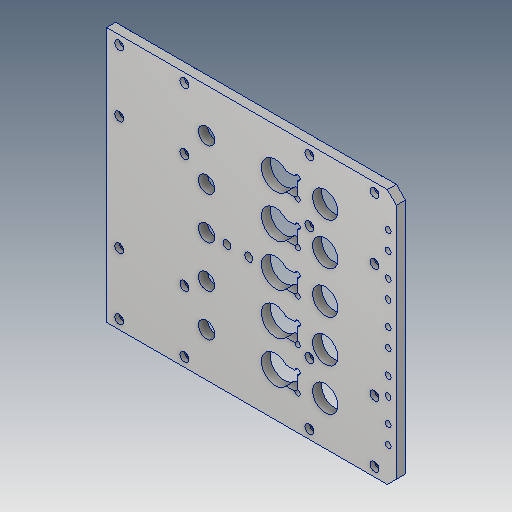
# Autodesk Inventor part: bottom-plate
Saved by Autodesk Inventor 2017 (Build 210142000, 142)
## iProperties
Created: 2018-06-17
Part Number: bottom-plate
Material: Aluminum 6061
Document SubType Name: Sheet Metal
Designer: Luiz Gustavo
Density: 2.7 g/cm^3
Sheet Metal Rule: Default_mm
Appearance: Aluminum - Flat
Author: Luiz Gustavo
Autodesk Inventor part; units mm, degrees
ref_plane "YZ Plane" through (0, 0, 0) normal (1, 0, 0) x (0, 1, 0)
ref_plane "XZ Plane" through (0, 0, 0) normal (0, 1, 0) x (-1, 0, 0)
ref_plane "XY Plane" through (0, 0, 0) normal (0, 0, 1) x (1, 0, 0)
sketch "Sketch1" plane through (0, 0, 0) normal (0, 0, 1) x (1, 0, 0)
  line L0 (-37.3, 70.5) -> (-32.3, 70.5) construction
  line L1 (-37.3, 52.15) -> (-37.3, 70.5) construction
  arc A0 (-37.3, 40.65) -> (-37.3, 52.15) centre (-37.3, 46.4) ccw construction
  line L2 (-37.3, 28.95) -> (-37.3, 40.65) construction
  arc A1 (-37.3, 17.45) -> (-37.3, 28.95) centre (-37.3, 23.2) ccw construction
  line L3 (-37.3, 5.75) -> (-37.3, 17.45) construction
  arc A2 (-37.3, -5.75) -> (-37.3, 5.75) centre (-37.3, 0) ccw construction
  line L4 (-37.3, -17.45) -> (-37.3, -5.75) construction
  arc A3 (-37.3, -28.95) -> (-37.3, -17.45) centre (-37.3, -23.2) ccw construction
  line L5 (-37.3, -40.65) -> (-37.3, -28.95) construction
  arc A4 (-37.3, -52.15) -> (-37.3, -40.65) centre (-37.3, -46.4) ccw construction
  line L6 (-37.3, -52.15) -> (-37.3, -70.5) construction
  line L7 (-37.3, -70.5) -> (-32.3, -70.5) construction
  circle A5 centre (24.95, -51.4) radius 2.05 construction
  circle A6 centre (24.95, -28.2) radius 2.05 construction
  circle A7 centre (24.95, -5) radius 2.05 construction
  circle A8 centre (24.95, 18.2) radius 2.05 construction
  circle A9 centre (24.95, 41.4) radius 2.05 construction
  line L8 (-23.6527, -42.9) -> (-20.4, -42.9) construction
  line L9 (-20.4, -42.9) -> (-20.4, -36.3) construction
  line L10 (-20.4, -36.3) -> (20.4, -36.3) construction
  line L11 (20.4, -36.3) -> (20.4, -56.5) construction
  line L12 (20.4, -56.5) -> (-20.4, -56.5) construction
  line L13 (-20.4, -56.5) -> (-20.4, -49.9) construction
  line L14 (-20.4, -49.9) -> (-23.6527, -49.9) construction
  arc A10 (-26.4473, -49.9) -> (-23.6527, -49.9) centre (-25.05, -51.4) ccw construction
  line L15 (-28.4, -49.9) -> (-28.4, -42.9) construction
  arc A11 (-23.6527, -42.9) -> (-26.4473, -42.9) centre (-25.05, -41.4) ccw construction
  line L16 (-23.6527, -19.7) -> (-20.4, -19.7) construction
  line L17 (-20.4, -19.7) -> (-20.4, -13.1) construction
  line L18 (-20.4, -13.1) -> (20.4, -13.1) construction
  line L19 (20.4, -13.1) -> (20.4, -33.3) construction
  line L20 (20.4, -33.3) -> (-20.4, -33.3) construction
  line L21 (-20.4, -33.3) -> (-20.4, -26.7) construction
  line L22 (-20.4, -26.7) -> (-23.6527, -26.7) construction
  arc A12 (-26.4473, -26.7) -> (-23.6527, -26.7) centre (-25.05, -28.2) ccw construction
  line L23 (-28.4, -26.7) -> (-28.4, -19.7) construction
  arc A13 (-23.6527, -19.7) -> (-26.4473, -19.7) centre (-25.05, -18.2) ccw construction
  line L24 (-23.6527, 3.5) -> (-20.4, 3.5) construction
  line L25 (-20.4, 3.5) -> (-20.4, 10.1) construction
  line L26 (-20.4, 10.1) -> (20.4, 10.1) construction
  line L27 (20.4, 10.1) -> (20.4, -10.1) construction
  line L28 (20.4, -10.1) -> (-20.4, -10.1) construction
  line L29 (-20.4, -10.1) -> (-20.4, -3.5) construction
  line L30 (-20.4, -3.5) -> (-23.6527, -3.5) construction
  arc A14 (-26.4473, -3.5) -> (-23.6527, -3.5) centre (-25.05, -5) ccw construction
  line L31 (-28.4, -3.5) -> (-28.4, 3.5) construction
  arc A15 (-23.6527, 3.5) -> (-26.4473, 3.5) centre (-25.05, 5) ccw construction
  line L32 (-23.6527, 26.7) -> (-20.4, 26.7) construction
  line L33 (-20.4, 26.7) -> (-20.4, 33.3) construction
  line L34 (-20.4, 33.3) -> (20.4, 33.3) construction
  line L35 (20.4, 33.3) -> (20.4, 13.1) construction
  line L36 (20.4, 13.1) -> (-20.4, 13.1) construction
  line L37 (-20.4, 13.1) -> (-20.4, 19.7) construction
  line L38 (-20.4, 19.7) -> (-23.6527, 19.7) construction
  arc A16 (-26.4473, 19.7) -> (-23.6527, 19.7) centre (-25.05, 18.2) ccw construction
  line L39 (-28.4, 19.7) -> (-28.4, 26.7) construction
  arc A17 (-23.6527, 26.7) -> (-26.4473, 26.7) centre (-25.05, 28.2) ccw construction
  line L40 (-23.6527, 49.9) -> (-20.4, 49.9) construction
  line L41 (-20.4, 49.9) -> (-20.4, 56.5) construction
  line L42 (-20.4, 56.5) -> (20.4, 56.5) construction
  line L43 (20.4, 56.5) -> (20.4, 36.3) construction
  line L44 (20.4, 36.3) -> (-20.4, 36.3) construction
  line L45 (-20.4, 36.3) -> (-20.4, 42.9) construction
  line L46 (-20.4, 42.9) -> (-23.6527, 42.9) construction
  arc A18 (-26.4473, 42.9) -> (-23.6527, 42.9) centre (-25.05, 41.4) ccw construction
  line L47 (-28.4, 42.9) -> (-28.4, 49.9) construction
  arc A19 (-23.6527, 49.9) -> (-26.4473, 49.9) centre (-25.05, 51.4) ccw construction
  circle A20 centre (24.95, 51.4) radius 2.05 construction
  circle A21 centre (24.95, 28.2) radius 2.05 construction
  circle A22 centre (24.95, 5) radius 2.05 construction
  circle A23 centre (24.95, -18.2) radius 2.05 construction
  circle A24 centre (24.95, -41.4) radius 2.05 construction
  line L48 (29.5, -70.5) -> (-130.5, -70.5)
  line L49 (-130.5, -70.5) -> (-130.5, 70.5)
  line L50 (-130.5, 70.5) -> (29.5, 70.5)
  line L51 (29.5, 70.5) -> (29.5, -70.5)
  circle A25 centre (24.95, -51.4) radius 1.65
  circle A26 centre (24.95, -41.4) radius 1.65
  circle A27 centre (24.95, -28.2) radius 1.65
  circle A28 centre (24.95, -18.2) radius 1.65
  circle A29 centre (24.95, -5) radius 1.65
  circle A30 centre (24.95, 5) radius 1.65
  circle A31 centre (24.95, 18.2) radius 1.65
  circle A32 centre (24.95, 28.2) radius 1.65
  circle A33 centre (24.95, 41.4) radius 1.65
  circle A34 centre (24.95, 51.4) radius 1.65
  circle A35 centre (-25.05, 51.4) radius 1.5
  circle A36 centre (-25.05, 41.4) radius 1.5
  circle A37 centre (-25.05, 28.2) radius 1.5
  circle A38 centre (-25.05, 18.2) radius 1.5
  circle A39 centre (-25.05, 5) radius 1.5
  circle A40 centre (-25.05, -5) radius 1.5
  circle A41 centre (-25.05, -18.2) radius 1.5
  circle A42 centre (-25.05, -28.2) radius 1.5
  circle A43 centre (-25.05, -51.4) radius 1.5
  circle A44 centre (-25.05, -41.4) radius 1.5
  circle A45 centre (-37.3, -46.4) radius 7.75
  circle A46 centre (-37.3, -23.2) radius 7.75
  circle A47 centre (-37.3, 0) radius 7.75
  circle A48 centre (-37.3, 23.2) radius 7.75
  circle A49 centre (-37.3, 46.4) radius 7.75
  line L52 (-37.3, -46.4) -> (-9.8, -46.4) construction
  circle A50 centre (-9.8, -46.4) radius 7
  line L53 (-37.3, 46.4) -> (-9.8, 46.4) construction
  line L54 (-9.8, 46.4) -> (-9.8, -46.4) construction
  line L55 (-37.3, 23.2) -> (-9.8, 23.2) construction
  line L56 (-37.3, -23.2) -> (-9.8, -23.2) construction
  line L57 (-37.3, 0) -> (-9.8, 0) construction
  circle A51 centre (-9.8, -23.2) radius 7
  circle A52 centre (-9.8, 0) radius 7
  circle A53 centre (-9.8, 23.2) radius 7
  circle A54 centre (-9.8, 46.4) radius 7
  circle A55 centre (-75.3, -46.4) radius 4.5
  line L58 (-37.3, -46.4) -> (-45.05, -46.4) construction
  line L59 (-37.3, 46.4) -> (-75.3, 46.4) construction
  line L60 (-75.3, 46.4) -> (-75.3, -46.4) construction
  line L61 (-37.3, -23.2) -> (-75.3, -23.2) construction
  line L62 (-37.3, 0) -> (-75.3, 0) construction
  line L63 (-37.3, 23.2) -> (-75.3, 23.2) construction
  circle A56 centre (-75.3, -23.2) radius 4.5
  circle A57 centre (-75.3, 0) radius 4.5
  circle A58 centre (-75.3, 23.2) radius 4.5
  circle A59 centre (-75.3, 46.4) radius 4.5
  line L64 (-45.05, -46.4) -> (-70.8, -46.4) construction
  line L65 (-70.8, -46.4) -> (-75.3, -46.4) construction
  circle A60 centre (-87.5161, -31.5337) radius 2.5 projected
  circle A61 centre (-87.5838, 31.2662) radius 2.5 projected
  circle A62 centre (-123.5838, 31.2274) radius 2.5 projected
  circle A63 centre (-123.5161, -31.5725) radius 2.5 projected
  arc A64 (-206.8064, -40.6623) -> (-200.7999, -46.6558) centre (-200.8064, -40.6558) ccw projected
  line L66 (-206.8064, -40.6623) -> (-206.8934, 40.1377) projected
  arc A65 (-200.8999, 46.1441) -> (-206.8934, 40.1377) centre (-200.8934, 40.1441) ccw projected
  line L67 (-40.4, 46.3171) -> (-200.8999, 46.1441) projected
  arc A66 (-40.4, 46.3171) -> (-34.4, 46.3235) centre (-37.4, 46.3203) ccw projected
  line L68 (-19.9, 46.3392) -> (-34.4, 46.3235) projected
  arc A67 (0.1, 46.3607) -> (-19.9, 46.3392) centre (-9.9, 46.3499) ccw projected
  line L69 (0.2, -46.4392) -> (0.1, 46.3607) projected
  arc A68 (-19.8, -46.4608) -> (0.2, -46.4392) centre (-9.8, -46.45) ccw projected
  line L70 (-19.8, -46.4608) -> (-34.3, -46.4764) projected
  arc A69 (-34.3, -46.4764) -> (-40.3, -46.4829) centre (-37.3, -46.4796) ccw projected
  line L71 (-40.3, -46.4829) -> (-200.7999, -46.6558) projected
  arc A70 (-190.8268, -21.6451) -> (-195.8268, -21.6504) centre (-193.3268, -21.6478) ccw projected
  line L72 (-195.8268, -21.6504) -> (-195.8161, -31.6504) projected
  arc A71 (-195.8161, -31.6504) -> (-190.8161, -31.6451) centre (-193.3161, -31.6477) ccw projected
  line L73 (-190.8161, -31.6451) -> (-190.8268, -21.6451) projected
  arc A72 (-190.8837, 31.1549) -> (-195.8837, 31.1495) centre (-193.3837, 31.1522) ccw projected
  line L74 (-195.8837, 31.1495) -> (-195.873, 21.1495) projected
  arc A73 (-195.873, 21.1495) -> (-190.873, 21.1549) centre (-193.373, 21.1522) ccw projected
  line L75 (-190.873, 21.1549) -> (-190.8837, 31.1549) projected
  arc A74 (-165.8837, 31.1819) -> (-170.8837, 31.1765) centre (-168.3837, 31.1792) ccw projected
  line L76 (-170.8837, 31.1765) -> (-170.873, 21.1765) projected
  arc A75 (-170.873, 21.1765) -> (-165.873, 21.1819) centre (-168.373, 21.1792) ccw projected
  line L77 (-165.873, 21.1819) -> (-165.8837, 31.1819) projected
  circle A76 centre (-37.375, 23.1203) radius 3 projected
  circle A77 centre (-37.325, -23.2796) radius 3 projected
  circle A78 centre (-37.35, -0.0797) radius 3 projected
  arc A79 (-178.373, 21.1684) -> (-183.373, 21.163) centre (-180.873, 21.1657) ccw projected
  line L78 (-183.373, 21.163) -> (-183.3622, 11.163) projected
  arc A80 (-183.3622, 11.163) -> (-178.3622, 11.1684) centre (-180.8622, 11.1657) ccw projected
  line L79 (-178.3622, 11.1684) -> (-178.373, 21.1684) projected
  arc A81 (-178.3376, -11.6316) -> (-183.3376, -11.637) centre (-180.8376, -11.6343) ccw projected
  line L80 (-183.3376, -11.637) -> (-183.3268, -21.637) projected
  arc A82 (-183.3268, -21.637) -> (-178.3268, -21.6316) centre (-180.8268, -21.6343) ccw projected
  line L81 (-178.3268, -21.6316) -> (-178.3376, -11.6316) projected
  arc A83 (-165.8268, -21.6181) -> (-170.8268, -21.6235) centre (-168.3268, -21.6208) ccw projected
  line L82 (-170.8268, -21.6235) -> (-170.8161, -31.6235) projected
  arc A84 (-170.8161, -31.6235) -> (-165.8161, -31.6181) centre (-168.3161, -31.6208) ccw projected
  line L83 (-165.8161, -31.6181) -> (-165.8268, -21.6181) projected
  circle A85 centre (-9.9, 46.3499) radius 1.1 projected
  circle A86 centre (-9.875, 23.15) radius 1.1 projected
  circle A87 centre (-9.8, -46.45) radius 1.1 projected
  circle A88 centre (-9.825, -23.25) radius 1.1 projected
  circle A89 centre (-9.85, -0.05) radius 1.1 projected
  line L84 (-26.4473, 42.9) -> (-28.4, 42.9) projected
  line L85 (-28.4, 49.9) -> (-26.4473, 49.9) projected
  line L86 (-26.4473, -3.5) -> (-28.4, -3.5) projected
  line L87 (-28.4, 3.5) -> (-26.4473, 3.5) projected
  line L88 (-26.4473, -49.9) -> (-28.4, -49.9) projected
  line L89 (-28.4, -42.9) -> (-26.4473, -42.9) projected
  line L90 (-26.4473, -26.7) -> (-28.4, -26.7) projected
  line L91 (-28.4, -19.7) -> (-26.4473, -19.7) projected
  line L92 (-26.4473, 19.7) -> (-28.4, 19.7) projected
  line L93 (-28.4, 26.7) -> (-26.4473, 26.7) projected
  line L94 (29, 61.5) -> (-23.3, 61.5) projected
  arc A90 (-32.3, 70.5) -> (-23.3, 61.5) centre (-23.3, 70.5) ccw projected
  arc A91 (-23.3, -61.5) -> (-32.3, -70.5) centre (-23.3, -70.5) ccw projected
  line L95 (-23.3, -61.5) -> (29, -61.5) projected
  line L96 (29, -61.5) -> (29, 61.5) projected
  point P0 (0, 0)
  dimension "d2" = 15.5
  dimension "d5" = 9
  dimension "d0" = 160
  dimension "d3" = 27.5
  dimension "d4" = 14
  dimension "d6" = 38
  dimension "d28" = 25.75
  dimension "d78" = 3
  dimension "d79" = 3.3
  constraints: 36 end point, 33 centre point, 28 equal radius, 24 coincident, 9 horizontal, 4 perpendicular, 4 point on line, 2 collinear, 2 horizontal alignment, 2 midpoint, 2 parallel, 1 vertical, 6 other
  measures "d0" distance between parallel lines of L49 L51
  measures "d3" distance of L52.start L52.end
  measures "d4" diameter of A50
  measures "d6" distance of L52.start L60.end
  measures "d28" distance of L58.end L64.end
  measures "d78" diameter of A35
  measures "d79" diameter of A34
extrude "Plate1" add sketch "Sketch1" along normal blind 5 contours L48 A91 L95 L96 L94 A90 L50 L51 | L48 L49 L71 A55 A45 L70 A68 L69 A67 L68 A49 L67 A59 L50 A90 L94 L96 L95 A91 | L49 L67 A59 A49 L68 A67 L69 A68 L70 A45 L71 A55 | A60 | A61 | A62 | A63
sketch "Sketch2" plane through (0, 0, 0) normal (0, 0, 1) x (1, 0, 0)
  line L0 (24.5, -70.5) -> (-25.5, -70.5) construction
  line L1 (-25.5, -70.5) -> (-25.5, -26.5) construction
  line L2 (-25.5, -26.5) -> (24.5, -26.5) construction
  line L3 (24.5, -26.5) -> (24.5, -70.5) construction
  circle A0 centre (-18.5, -65.5) radius 2.5
  circle A1 centre (17.5, -65.5) radius 2.5
  circle A2 centre (17.5, -31.5) radius 2.5
  circle A3 centre (-18.5, -31.5) radius 2.5
  line L4 (-18.5, -65.5) -> (17.5, -65.5) construction
  line L5 (17.5, -65.5) -> (17.5, -31.5) construction
  line L6 (17.5, -31.5) -> (-18.5, -31.5) construction
  line L7 (-18.5, -31.5) -> (-18.5, -65.5) construction
  line L8 (-12.7, -31.5) -> (-12.7, -65.5) construction
  line L9 (11.7, -31.5) -> (11.7, -65.5) construction
  line L10 (29.5, -70.5) -> (-130.5, -70.5) construction
  line L11 (-130.5, -70.5) -> (-130.5, 70.5) construction
  line L12 (29.5, 70.5) -> (29.5, -70.5) construction
  line L13 (-130.5, 70.5) -> (29.5, 70.5) construction
  line L14 (-80.5, -70.5) -> (-130.5, -70.5) construction
  line L15 (-130.5, -70.5) -> (-130.5, -26.5) construction
  line L16 (-130.5, -26.5) -> (-80.5, -26.5) construction
  line L17 (-80.5, -26.5) -> (-80.5, -70.5) construction
  circle A4 centre (-123.5, -65.5) radius 2.5
  circle A5 centre (-87.5, -65.5) radius 2.5
  circle A6 centre (-87.5, -31.5) radius 2.5
  circle A7 centre (-123.5, -31.5) radius 2.5
  line L18 (-123.5, -65.5) -> (-87.5, -65.5) construction
  line L19 (-87.5, -65.5) -> (-87.5, -31.5) construction
  line L20 (-87.5, -31.5) -> (-123.5, -31.5) construction
  line L21 (-123.5, -31.5) -> (-123.5, -65.5) construction
  line L22 (-117.7, -31.5) -> (-117.7, -65.5) construction
  line L23 (-93.3, -31.5) -> (-93.3, -65.5) construction
  line L24 (-123.5, 31.5) -> (-87.5, 31.5) construction
  line L25 (-87.5, 65.5) -> (-123.5, 65.5) construction
  line L26 (-130.5, 70.5) -> (-80.5, 70.5) construction
  line L27 (-117.7, 65.5) -> (-117.7, 31.5) construction
  line L28 (-123.5, 65.5) -> (-123.5, 31.5) construction
  circle A8 centre (-123.5, 65.5) radius 2.5
  line L29 (-130.5, 26.5) -> (-130.5, 70.5) construction
  circle A9 centre (-123.5, 31.5) radius 2.5
  line L30 (-93.3, 65.5) -> (-93.3, 31.5) construction
  circle A10 centre (-87.5, 31.5) radius 2.5
  line L31 (-87.5, 31.5) -> (-87.5, 65.5) construction
  circle A11 centre (-87.5, 65.5) radius 2.5
  line L32 (-80.5, 70.5) -> (-80.5, 26.5) construction
  line L33 (-80.5, 26.5) -> (-130.5, 26.5) construction
  line L34 (-18.5, 31.5) -> (17.5, 31.5) construction
  line L35 (17.5, 65.5) -> (-18.5, 65.5) construction
  line L36 (-25.5, 70.5) -> (24.5, 70.5) construction
  line L37 (-12.7, 65.5) -> (-12.7, 31.5) construction
  line L38 (-18.5, 65.5) -> (-18.5, 31.5) construction
  circle A12 centre (-18.5, 65.5) radius 2.5
  line L39 (-25.5, 26.5) -> (-25.5, 70.5) construction
  circle A13 centre (-18.5, 31.5) radius 2.5
  line L40 (11.7, 65.5) -> (11.7, 31.5) construction
  circle A14 centre (17.5, 31.5) radius 2.5
  line L41 (17.5, 31.5) -> (17.5, 65.5) construction
  circle A15 centre (17.5, 65.5) radius 2.5
  line L42 (24.5, 70.5) -> (24.5, 26.5) construction
  line L43 (24.5, 26.5) -> (-25.5, 26.5) construction
  point P0 (0, 0)
  dimension "d8" = 44
  dimension "d9" = 50
  dimension "d10" = 5
  dimension "d11" = 5
  dimension "d12" = 7
  dimension "d13" = 5
  dimension "d14" = 7
  dimension "d15" = 24.4
  dimension "d16" = 12.8
  dimension "d17" = 0
  dimension "d18" = 5
  dimension "d19" = 44
  dimension "d20" = 50
  dimension "d21" = 5
  dimension "d22" = 5
  dimension "d23" = 7
  dimension "d24" = 5
  dimension "d25" = 7
  dimension "d26" = 24.4
  dimension "d27" = 12.8
  dimension "d30" = 0
  dimension "d31" = 0
  dimension "d32" = 44
  dimension "d33" = 50
  dimension "d34" = 5
  dimension "d35" = 5
  dimension "d36" = 7
  dimension "d37" = 5
  dimension "d38" = 7
  dimension "d39" = 24.4
  dimension "d40" = 12.8
  dimension "d41" = 44
  dimension "d42" = 50
  dimension "d43" = 5
  dimension "d44" = 5
  dimension "d45" = 7
  dimension "d46" = 5
  dimension "d47" = 7
  dimension "d48" = 24.4
  dimension "d49" = 12.8
  dimension "d50" = 0
  dimension "d51" = 0
  dimension "d52" = 5
  dimension "d53" = 0
  constraints: 80 end point, 20 parallel, 16 centre point, 16 point on line, 12 coincident, 12 equal radius, 12 perpendicular, 8 horizontal
  measures "d8" distance of L2.end L0.start
  measures "d9" distance between parallel lines of L1 L3
  measures "d10" diameter of A0
  measures "d11" distance between parallel lines of L4 L0
  measures "d12" distance between parallel lines of L1 L7
  measures "d13" distance between parallel lines of L2 L6
  measures "d14" distance between parallel lines of L3 L5
  measures "d15" distance between parallel lines of L9 L8
  measures "d16" distance between parallel lines of L1 L8
  measures "d17" distance between parallel lines of L10 L0
  measures "d18" distance between parallel lines of L12 L3
  measures "d19" distance of L16.end L17.end
  measures "d20" distance between parallel lines of L15 L17
  measures "d21" diameter of A4
  measures "d22" distance between parallel lines of L18 L14
  measures "d23" distance between parallel lines of L15 L21
  measures "d24" distance between parallel lines of L16 L20
  measures "d25" distance between parallel lines of L17 L19
  measures "d26" distance between parallel lines of L23 L22
  measures "d27" distance between parallel lines of L15 L22
  measures "d30" distance between parallel lines of L10 L14
  measures "d31" distance between parallel lines of L11 L15
  measures "d32" distance of L26.end L33.start
  measures "d33" distance between parallel lines of L29 L32
  measures "d34" diameter of A9
  measures "d35" distance between parallel lines of L24 L33
  measures "d36" distance between parallel lines of L29 L28
  measures "d37" distance between parallel lines of L26 L25
  measures "d38" distance between parallel lines of L32 L31
  measures "d39" distance between parallel lines of L30 L27
  measures "d40" distance between parallel lines of L29 L27
  measures "d41" distance of L36.end L43.start
  measures "d42" distance between parallel lines of L39 L42
  measures "d43" diameter of A13
  measures "d44" distance between parallel lines of L34 L43
  measures "d45" distance between parallel lines of L39 L38
  measures "d46" distance between parallel lines of L36 L35
  measures "d47" distance between parallel lines of L42 L41
  measures "d48" distance between parallel lines of L40 L37
  measures "d49" distance between parallel lines of L39 L37
  measures "d50" distance between parallel lines of L26 L13
  measures "d51" distance between parallel lines of L11 L29
  measures "d52" distance between parallel lines of L12 L42
  measures "d53" distance between parallel lines of L13 L36
hole "Hole1" at (-123.5, 65.5, 0) at (-123.5, 31.5, 0) at (-87.5, 65.5, 0) at (-87.5, 31.5, 0) at (-123.5, -31.5, 0) at (-123.5, -65.5, 0) at (-87.5, -65.5, 0) at (-87.5, -31.5, 0) at (-18.5, -65.5, 0) at (17.5, -65.5, 0) at (17.5, -31.5, 0) at (-18.5, -31.5, 0) at (-18.5, 31.5, 0) at (-18.5, 65.5, 0) at (17.5, 65.5, 0) at (17.5, 31.5, 0) direction (0, 0, 1) diameter 5 end through all countersink diameter 10 countersink angle 90
sketch "Sketch3" plane through (0, 0, 0) normal (0, 0, 1) x (1, 0, 0)
  line L0 (-47.5, -20) -> (-56.5, -20)
  line L1 (-56.5, -20) -> (-56.5, 20)
  line L2 (-56.5, 20) -> (-47.5, 20)
  line L3 (-47.5, 20) -> (-47.5, -20)
  line L4 (-59.5, 20) -> (-68.5, 20)
  line L5 (-68.5, 20) -> (-68.5, -20)
  line L6 (-68.5, -20) -> (-59.5, -20)
  line L7 (-59.5, -20) -> (-59.5, 20)
  line L8 (-47.5, 0) -> (-68.5, 0) construction
  line L9 (-64, 20) -> (-64, -20) construction
  line L10 (-52, 20) -> (-52, -20) construction
  circle A0 centre (-64, 0) radius 2
  circle A1 centre (-52, 0) radius 2
  line L11 (-130.5, 70.5) -> (29.5, 70.5) projected
  line L12 (-130.5, -70.5) -> (-130.5, 70.5) projected
  line L13 (29.5, -70.5) -> (-130.5, -70.5) projected
  line L14 (-130.5, 0) -> (-68.5, 0) construction
  point P0 (0, 0)
  dimension "d61" = 9
  dimension "d62" = 40
  dimension "d63" = 3
  dimension "d64" = 4
  dimension "d65" = 62
  constraints: 24 end point, 9 midpoint, 4 parallel, 3 collinear, 3 horizontal, 2 centre point, 2 perpendicular, 1 equal radius
  measures "d61" distance of L1.end L2.end
  measures "d62" distance between parallel lines of L0 L2
  measures "d63" distance between parallel lines of L1 L7
  measures "d64" diameter of A0
  measures "d65" distance between parallel lines of L12 L5
hole "Hole2" at (-52, 0, 0) at (-64, 0, 0) direction (0, 0, 1) diameter 4.5 end through all
sketch "Sketch4" plane through (0, 0, 0) normal (0, 0, 1) x (1, 0, 0)
  circle A0 centre (-25.05, -41.4) radius 1.5 projected
  circle A1 centre (-25.05, -51.4) radius 1.5 projected
  circle A2 centre (-37.3, -46.4) radius 7.75 projected
  circle A3 centre (-25.05, -28.2) radius 1.5 projected
  circle A4 centre (-37.3, -23.2) radius 7.75 projected
  circle A5 centre (-25.05, -18.2) radius 1.5 projected
  circle A6 centre (-25.05, -5) radius 1.5 projected
  circle A7 centre (-37.3, 0) radius 7.75 projected
  circle A8 centre (-25.05, 5) radius 1.5 projected
  circle A9 centre (-25.05, 18.2) radius 1.5 projected
  circle A10 centre (-37.3, 23.2) radius 7.75 projected
  circle A11 centre (-25.05, 28.2) radius 1.5 projected
  circle A12 centre (-25.05, 41.4) radius 1.5 projected
  circle A13 centre (-37.3, 46.4) radius 7.75 projected
  circle A14 centre (-25.05, 51.4) radius 1.5 projected
  line L0 (-25.05, -41.4) -> (-37.3, -41.4)
  line L1 (-37.3, -41.4) -> (-37.3, -51.4)
  line L2 (-37.3, -51.4) -> (-25.05, -51.4)
  line L3 (-25.05, -51.4) -> (-25.05, -41.4)
  line L4 (-25.05, -18.2) -> (-37.3, -18.2)
  line L5 (-37.3, -18.2) -> (-37.3, -28.2)
  line L6 (-37.3, -28.2) -> (-25.05, -28.2)
  line L7 (-25.05, -28.2) -> (-25.05, -18.2)
  line L8 (-25.05, 5) -> (-37.3, 5)
  line L9 (-37.3, 5) -> (-37.3, -5)
  line L10 (-37.3, -5) -> (-25.05, -5)
  line L11 (-25.05, -5) -> (-25.05, 5)
  line L12 (-25.05, 28.2) -> (-37.3, 28.2)
  line L13 (-37.3, 28.2) -> (-37.3, 18.2)
  line L14 (-37.3, 18.2) -> (-25.05, 18.2)
  line L15 (-25.05, 18.2) -> (-25.05, 28.2)
  line L16 (-25.05, 51.4) -> (-37.3, 51.4)
  line L17 (-37.3, 51.4) -> (-37.3, 41.4)
  line L18 (-37.3, 41.4) -> (-25.05, 41.4)
  line L19 (-25.05, 41.4) -> (-25.05, 51.4)
  point P0 (0, 0)
  constraints: 40 end point, 10 parallel, 7 coincident, 5 horizontal, 5 midpoint, 5 perpendicular
extrude "Cut1" cut sketch "Sketch4" along normal blind 5 contours L0 L3 A0 | A0 L3 A1 L2 A2 L0 | A2 L2 L1 L0 | L3 L2 A1 | L7 L6 A3 | A3 L6 A4 L4 A5 L7 | A5 L4 L7 | L6 L5 L4 A4 | L11 L10 A6 | A6 L10 A7 L8 A8 L11 | A8 L8 L11 | L10 L9 L8 A7 | L15 L14 A9 | A9 L14 A10 L12 A11 L15 | A11 L12 L15 | L14 L13 L12 A10 | L19 L18 A12 | A12 L18 A13 L16 A14 L19 | A14 L16 L19 | L18 L17 L16 A13 picked at (-26.0375, -41.5113) picked at (-34.7167, -46.4) picked at (-25.8914, -50.8713) picked at (-25.9879, -27.8718) picked at (-26.0375, -18.3113) picked at (-34.7167, -23.2) picked at (-25.3782, -4.0621) picked at (-26.0375, 4.8887) picked at (-34.7167, 0) picked at (-25.9879, 18.5282) picked at (-26.0375, 28.0887) picked at (-34.7167, 23.2) picked at (-25.8914, 41.9287) picked at (-26.0375, 51.2887) picked at (-34.7167, 46.4)
chamfer "Corner Chamfer1" distance 5 angle 45 2 edges at (29.5, -70.5, 2.5) (29.5, 70.5, 2.5)
equation "\"d13\" = d11"
equation "\"d14\" = d12"
equation "\"d24\" = d22"
equation "\"d25\" = d23"
equation "\"d37\" = d35"
equation "\"d38\" = d36"
equation "\"d46\" = d44"
equation "\"d47\" = d45"
equation "\"d59\" = Thickness"
equation "\"d71\" = Thickness"
equation "\"d73\" = Thickness"
equation "\"BendRadius\" = Thickness"
equation "\"BendReliefWidth\" = Thickness"
equation "\"BendReliefDepth\" = 0.5 * Thickness"
equation "\"TransitionRadius\" = BendRadius"
equation "\"JacobiRadiusSize\" = BendRadius"
equation "\"GapSize\" = Thickness"
equation "\"d7\" = BendRadius"
equation "\"Thickness\" = 5"
body "Solid1"
